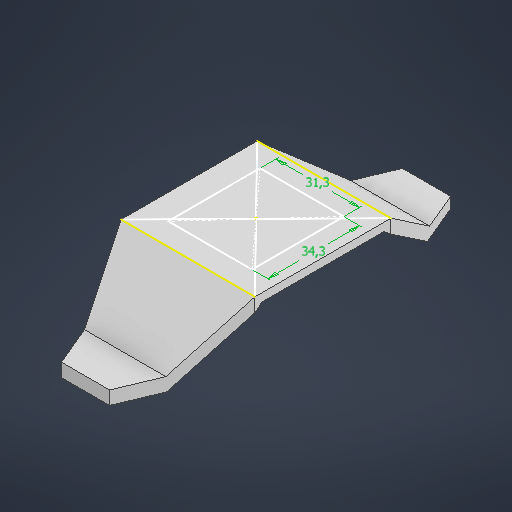
# Autodesk Inventor part: Деталь1
Saved by Autodesk Inventor 2026.2 (Build 302298000, 298)
## iProperties
Created: 2026-01-23
Part Number: Деталь1
Material: Типовые
Document SubType Name: Modeling
Designer: Phantom
Density: 1 g/cm^3
Appearance: По умолчанию
Author: Phantom
Autodesk Inventor part; units mm, degrees
ref_plane "YZ Plane" through (0, 0, 0) normal (1, 0, 0) x (0, 1, 0)
ref_plane "XZ Plane" through (0, 0, 0) normal (0, 1, 0) x (-1, 0, 0)
ref_plane "XY Plane" through (0, 0, 0) normal (0, 0, 1) x (1, 0, 0)
sketch "Эскиз1" plane through (0, 0, 0) normal (0, 1, 0) x (-1, 0, 0)
  line L0 (-25, 22.7625) -> (25, 22.7625)
  line L1 (25, 22.7625) -> (25, -22.7625)
  line L2 (25, -22.7625) -> (-25, -22.7625)
  line L3 (-25, -22.7625) -> (-25, 22.7625)
  line L4 (-25, 22.7625) -> (25, -22.7625) construction
  line L5 (25, 22.7625) -> (-25, -22.7625) construction
  point P0 (0, 0)
  dimension "d0" = 50
  dimension "d1" = 45.525
  constraints: 12 end point, 2 midpoint, 2 parallel, 1 horizontal, 1 perpendicular
  measures "d0" distance of L1.end L2.end
  measures "d1" distance of L0.end L1.end
extrude "Выдавливание1" add sketch "Эскиз1" along normal blind 3
sketch "Эскиз3" plane through (25, 0, 22.7625) normal (1, 0, 0) x (0, 0, -1)
  line L0 (45.525, 0) -> (0, 0) projected
  line L1 (0, 0) -> (0, -21)
  line L2 (45.525, 3) -> (0, 3) projected
  line L3 (0, -21) -> (-43.1562, -21)
  line L4 (0, -21) -> (135.6288, -21)
  line L5 (0, 0) -> (-25.9328, -21)
  line L6 (45.525, 0) -> (71.4578, -21)
  line L7 (71.4578, -21) -> (86.4578, -21)
  line L8 (86.4578, -21) -> (86.4578, -17)
  line L9 (86.4578, -17) -> (72.8743, -17)
  line L10 (-25.9328, -21) -> (-40.9328, -21)
  line L11 (-40.9328, -21) -> (-40.9328, -16)
  line L12 (-40.9328, -16) -> (-26.1144, -16)
  line L13 (-2.6514, 3) -> (-26.1144, -16)
  line L14 (0, 3) -> (-2.6514, 3)
  line L15 (48.1764, 3) -> (72.8743, -17)
  line L16 (45.525, 3) -> (48.1764, 3)
  line L17 (0, 3) -> (0, 0)
  line L18 (45.525, 0) -> (45.525, 3) projected
  line L19 (45.525, 3) -> (45.525, 0)
  line L20 (45.525, 3) -> (45.525, 0)
  point P0 (22.7625, 0)
  dimension "d4" = 21
  dimension "d7" = 15
  dimension "d8" = 4
  dimension "d9" = 15
  dimension "d10" = 5
  dimension "d11" = 4
  dimension "d12" = 4
  constraints: 36 end point, 5 perpendicular, 4 horizontal, 4 point on line, 2 parallel, 2 vertical, 1 collinear
  measures "d4" distance of L0.end L1.end
  measures "d7" distance of L6.end L7.end
  measures "d8" distance of L7.end L8.end
  measures "d9" distance of L5.end L10.end
  measures "d10" distance of L10.end L11.end
  measures "d11" distance between parallel lines of L5 L13
  measures "d12" distance between parallel lines of L6 L15
extrude "Выдавливание2" add sketch "Эскиз3" against normal up to surface (50 mm away) contours L18 L16 L15 L9 L8 L4 L6 | L5 L3 L11 L12 L13 L14 L17
sketch "Эскиз4" plane through (25, -16, 63.6953) normal (0, 1, 0) x (1, 0, 0)
  line L0 (0, 89.1092) -> (0, 38.2815) projected
  line L1 (0, 38.2815) -> (-16, 0)
  line L2 (0, 0) -> (-50, 0) projected
  line L3 (-50, 38.2815) -> (-50, 14.8184) projected
  line L4 (-50, 38.2815) -> (-34, 0)
  line L5 (-50, 14.8184) -> (-50, 0) projected
  line L6 (0, 14.8184) -> (0, 0) projected
  line L7 (-16, 0) -> (0, 0)
  line L8 (0, 38.2815) -> (0, 0)
  line L9 (-34, 0) -> (-50, 0)
  line L10 (-50, 0) -> (-50, 38.2815)
  point P0 (-25, 63.6953)
  dimension "d15" = 16
  dimension "d16" = 16
  constraints: 12 end point, 2 collinear, 2 point on line, 1 horizontal, 1 perpendicular
  measures "d15" distance from line of L5 L4.end
  measures "d16" distance from line of L6 L1.end
extrude "Выдавливание3" cut sketch "Эскиз4" along normal mid plane 70
sketch "Эскиз5" plane through (0, 3, 0) normal (0, 1, 0) x (1, 0, 0)
  line L0 (-15.1935, -48.8769) -> (-9, -63.6953) projected
  line L1 (-25, 25.4139) -> (-25, -25.4139) projected
  line L2 (-25, 25.4139) -> (-9, 63.6953)
  line L3 (25, 63.6953) -> (-25, 63.6953) projected
  line L4 (25, 63.6953) -> (25, 50.1118) projected
  line L5 (25, 25.4139) -> (9.06, 63.6953)
  line L6 (-25, 25.4139) -> (-25, 63.6953)
  line L7 (-9, 63.6953) -> (-25, 63.6953)
  line L8 (25, 25.4139) -> (25, 63.6953)
  line L9 (25, 63.6953) -> (9.06, 63.6953)
  point P0 (0, 0)
  constraints: 12 end point, 2 collinear, 2 perpendicular, 1 point on line
extrude "Выдавливание4" cut sketch "Эскиз5" against normal blind 70
sketch "Эскиз7" plane through (0, 3, 0) normal (0, 1, 0) x (1, 0, 0)
  line L0 (25, -25.4139) -> (-25, -25.4139) projected
  line L1 (25, 25.4139) -> (-25, 25.4139) projected
  line L2 (-25, -25.4139) -> (25, 25.4139)
  line L3 (-25, 25.4139) -> (25, -25.4139)
  line L4 (-15.65, -17.15) -> (15.65, -17.15)
  line L5 (15.65, -17.15) -> (15.65, 17.15)
  line L6 (15.65, 17.15) -> (-15.65, 17.15)
  line L7 (-15.65, 17.15) -> (-15.65, -17.15)
  line L8 (-15.65, -17.15) -> (15.65, 17.15) construction
  line L9 (15.65, -17.15) -> (-15.65, 17.15) construction
  point P0 (0, 0)
  dimension "d21" = 31.3
  dimension "d22" = 34.3
  constraints: 16 end point, 2 midpoint, 2 parallel, 1 horizontal, 1 perpendicular
  measures "d21" distance of L6.end L5.end
  measures "d22" distance of L5.end L4.end
